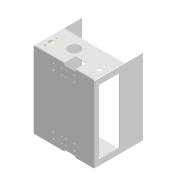
# Autodesk Inventor part: Part75
Saved by Autodesk Inventor 2020.5 (Build 245400000, 400)
## iProperties
Created: 2022-11-22
Part Number: Part75
Material: 一般
Document SubType Name: Sheet Metal
Designer: Administrator
Density: 1 g/cm^3
Appearance: 既定
Sheet Metal Rule: Default_mm
Author: Administrator
Autodesk Inventor part; units mm, degrees
ref_plane "YZ Plane" through (0, 0, 0) normal (1, 0, 0) x (0, 1, 0)
ref_plane "XZ Plane" through (0, 0, 0) normal (0, 1, 0) x (-1, 0, 0)
ref_plane "XY Plane" through (0, 0, 0) normal (0, 0, 1) x (1, 0, 0)
sketch "スケッチ1" plane through (0, 0, 0) normal (0, 0, 1) x (1, 0, 0)
  line L0 (28.4497, -88.6) -> (28.4497, -86) projected
  line L1 (28.4497, -86) -> (31.4997, -86) projected
  line L2 (31.5, -45.4) -> (31.4997, -86) projected
  line L3 (2, -45.3998) -> (31.5, -45.4) projected
  line L4 (2, -45.3998) -> (1.9997, -85.9998) projected
  line L5 (1.9997, -85.9998) -> (5.0497, -85.9998) projected
  line L6 (5.0497, -85.9998) -> (5.0497, -88.5998) projected
  line L7 (28.4497, -88.6) -> (5.0497, -88.5998) projected
  circle A0 centre (27.9998, -75) radius 1.35 projected
  circle A1 centre (5.4999, -58.9999) radius 1.35 projected
  circle A2 centre (5.4998, -74.9999) radius 1.35 projected
  circle A3 centre (27.9999, -59) radius 1.35 projected
  line L8 (38.5497, -88.6) -> (61.9497, -88.6002) projected
  line L9 (61.9497, -86.0002) -> (61.9497, -88.6002) projected
  line L10 (64.9997, -86.0002) -> (61.9497, -86.0002) projected
  line L11 (65, -45.4002) -> (64.9997, -86.0002) projected
  line L12 (65, -45.4002) -> (35.5, -45.4) projected
  line L13 (35.5, -45.4) -> (35.4997, -86) projected
  line L14 (38.5497, -86) -> (35.4997, -86) projected
  line L15 (38.5497, -88.6) -> (38.5497, -86) projected
  circle A4 centre (61.4999, -59.0001) radius 1.35 projected
  circle A5 centre (38.9998, -75) radius 1.35 projected
  circle A6 centre (61.4998, -75.0001) radius 1.35 projected
  circle A7 centre (38.9999, -59) radius 1.35 projected
  line L16 (28.4492, -179.4) -> (28.4492, -182) projected
  line L17 (28.4492, -179.4) -> (5.0492, -179.3998) projected
  line L18 (5.0492, -181.9998) -> (5.0492, -179.3998) projected
  line L19 (1.9992, -181.9998) -> (5.0492, -181.9998) projected
  line L20 (1.999, -222.5998) -> (1.9992, -181.9998) projected
  line L21 (1.999, -222.5998) -> (31.499, -222.6) projected
  line L22 (31.499, -222.6) -> (31.4992, -182) projected
  line L23 (28.4492, -182) -> (31.4992, -182) projected
  circle A8 centre (27.9992, -193) radius 1.35 projected
  circle A9 centre (5.4991, -208.9999) radius 1.35 projected
  circle A10 centre (5.4992, -192.9999) radius 1.35 projected
  circle A11 centre (27.9991, -209) radius 1.35 projected
  line L24 (38.5492, -179.4) -> (61.9492, -179.4002) projected
  line L25 (38.5492, -179.4) -> (38.5492, -182) projected
  line L26 (38.5492, -182) -> (35.4992, -182) projected
  line L27 (35.499, -222.6) -> (35.4992, -182) projected
  line L28 (64.999, -222.6002) -> (35.499, -222.6) projected
  line L29 (64.999, -222.6002) -> (64.9992, -182.0002) projected
  line L30 (64.9992, -182.0002) -> (61.9492, -182.0002) projected
  line L31 (61.9492, -182.0002) -> (61.9492, -179.4002) projected
  circle A12 centre (61.4991, -209.0001) radius 1.35 projected
  circle A13 centre (38.9992, -193) radius 1.35 projected
  circle A14 centre (61.4992, -193.0001) radius 1.35 projected
  circle A15 centre (38.9991, -209) radius 1.35 projected
  line L32 (-44.591, -44.9996) -> (-44.5911, -55.9996) projected
  line L33 (-44.592, -222.9996) -> (-44.5919, -211.9996) projected
  line L34 (111.59, -223.0004) -> (111.5901, -213.0004) projected
  line L35 (111.591, -45.0004) -> (111.5909, -55.0004) projected
  circle A16 centre (61.4992, -193.0001) radius 1.6
  circle A17 centre (61.4991, -209.0001) radius 1.6
  circle A18 centre (38.9992, -193) radius 1.6
  circle A19 centre (38.9991, -209) radius 1.6
  circle A20 centre (27.9992, -193) radius 1.6
  circle A21 centre (27.9991, -209) radius 1.6
  circle A22 centre (5.4991, -208.9999) radius 1.6
  circle A23 centre (5.4992, -192.9999) radius 1.6
  line L36 (-46.4999, -223.01) -> (113.4979, -223.01)
  line L37 (113.4979, -223.01) -> (-46.5009, -223.01)
  line L38 (61.9497, -88.6002) -> (61.9497, -86.0002) projected
  line L39 (61.9497, -88.6002) -> (38.5497, -88.6) projected
  line L40 (38.5497, -86) -> (38.5497, -88.6) projected
  line L41 (35.4997, -86) -> (38.5497, -86) projected
  line L42 (35.5, -45.4) -> (35.4997, -86) projected
  line L43 (35.5, -45.4) -> (65, -45.4002) projected
  line L44 (65, -45.4002) -> (64.9997, -86.0002) projected
  line L45 (61.9497, -86.0002) -> (64.9997, -86.0002) projected
  circle A24 centre (61.4998, -75.0001) radius 1.35 projected
  circle A25 centre (38.9999, -59) radius 1.35 projected
  circle A26 centre (38.9998, -75) radius 1.35 projected
  circle A27 centre (61.4999, -59.0001) radius 1.35 projected
  line L46 (5.0497, -88.5998) -> (28.4497, -88.6) projected
  line L47 (5.0497, -88.5998) -> (5.0497, -85.9998) projected
  line L48 (5.0497, -85.9998) -> (1.9997, -85.9998) projected
  line L49 (2, -45.3998) -> (1.9997, -85.9998) projected
  line L50 (31.5, -45.4) -> (2, -45.3998) projected
  line L51 (31.5, -45.4) -> (31.4997, -86) projected
  line L52 (31.4997, -86) -> (28.4497, -86) projected
  line L53 (28.4497, -86) -> (28.4497, -88.6) projected
  circle A28 centre (27.9999, -59) radius 1.35 projected
  circle A29 centre (5.4998, -74.9999) radius 1.35 projected
  circle A30 centre (27.9998, -75) radius 1.35 projected
  circle A31 centre (5.4999, -58.9999) radius 1.35 projected
  line L54 (35.499, -222.6) -> (113.499, -222.6)
  line L55 (113.499, -222.6) -> (113.499, -45.4)
  line L56 (113.499, -45.4) -> (35.499, -45.4)
  line L57 (35.499, -45.4) -> (35.499, -222.6)
  line L58 (31.499, -222.6) -> (-46.5009, -222.6)
  line L59 (-46.5009, -222.6) -> (-46.5009, -45.4)
  line L60 (-46.5009, -45.4) -> (31.499, -45.4)
  line L61 (31.499, -45.4) -> (31.499, -222.6)
  line L62 (113.499, -45.4) -> (-46.5009, -45.4)
  circle A32 centre (61.4998, -75.0001) radius 1.6
  circle A33 centre (38.9998, -75) radius 1.6
  circle A34 centre (27.9998, -75) radius 1.6
  circle A35 centre (5.4998, -74.9999) radius 1.6
  circle A36 centre (61.4999, -59.0001) radius 1.6
  circle A37 centre (38.9999, -59) radius 1.6
  circle A38 centre (27.9999, -59) radius 1.6
  dimension "d4" = 78
  dimension "d5" = 78
  dimension "d14" = 3.2
  dimension "d15" = 3.2
  dimension "d16" = 3.2
  dimension "d17" = 3.2
  dimension "d18" = 3.2
  dimension "d19" = 3.2
  dimension "d20" = 3.2
  dimension "d21" = 3.2
  dimension "d99" = 78
  dimension "d100" = 3.2
  dimension "d101" = 3.2
  dimension "d102" = 3.2
  dimension "d103" = 3.2
  dimension "d104" = 3.2
  dimension "d105" = 3.2
  dimension "d106" = 3.2
  constraints: 22 end point, 15 centre point, 15 coincident, 4 horizontal, 4 parallel, 2 perpendicular, 1 collinear, 1 point on line
  measures "d4" distance of L27.start L36.end
  measures "d5" distance of L21.end L36.start
  measures "d14" diameter of A16
  measures "d15" diameter of A17
  measures "d16" diameter of A18
  measures "d17" diameter of A19
  measures "d18" diameter of A20
  measures "d19" diameter of A21
  measures "d20" diameter of A22
  measures "d21" diameter of A23
  measures "d99" distance of L56.end L55.end
  measures "d100" diameter of A32
  measures "d101" diameter of A33
  measures "d102" diameter of A34
  measures "d103" diameter of A35
  measures "d104" diameter of A36
  measures "d105" diameter of A37
  measures "d106" diameter of A38
sketch "スケッチ2" plane through (0, 0, 0) normal (0, 1, 0) x (-1, 0, 0)
  point P0 (0, 0)
extrude "押し出し1" add sketch "スケッチ1" along normal blind 1 contours L7 L6 L5 L4 L3 L2 L1 L0 | A0 | A1 | A2 | A3 | L15 L14 L13 L12 L11 L10 L9 L8 | A4 | A5 | A6 | A7 | A32 | A33 | A34 | A35 | A36 | A37 | A38
ref_plane "作業平面1" through (-47.4989, -223.01, -128) normal (-1, -0.0000053, 0) x (0, 0, 1)
sketch "スケッチ8" plane through (-47.4989, -223.01, -128) normal (-1, -0.0000053, 0) x (0, 0, 1)
  line L0 (69.5, 180.01) -> (69.5, 30.01) projected
  line L1 (69.5, 30.01) -> (109.5, 30.01) projected
  line L2 (109.5, 180.01) -> (109.5, 30.01) projected
  line L3 (69.5, 180.01) -> (109.5, 180.01) projected
  line L4 (0, 202.61) -> (127, 202.61) projected
  line L5 (127, 0) -> (0, 0) projected
  ellipse E0 centre (98, 9.01) end of major axis (109, 9.01) minor radius 0.0001 projected
  line L6 (62, 15) -> (117, 15)
  line L7 (117, 15) -> (117, 187.61)
  line L8 (117, 187.61) -> (62, 187.61)
  line L9 (62, 187.61) -> (62, 15)
  line L10 (127, 1) -> (127, 201.61) projected
  point P0 (128, 223.0098)
  dimension "d72" = 55
  dimension "d74" = 202.61
  dimension "d75" = 15
  dimension "d76" = 10
  dimension "d85" = 15
  constraints: 8 end point, 2 parallel, 1 horizontal, 1 perpendicular
  measures "d72" distance of L8.end L7.end
  measures "d74" distance between parallel lines of L4 L5
  measures "d75" distance between parallel lines of L6 L5
  measures "d76" distance between parallel lines of L10 L7
  measures "d85" distance between parallel lines of L4 L8
extrude "押し出し3" cut sketch "スケッチ8" against normal through all both and the other way through all contours L3 L2 L1 L0 | L9 L8 L7 L6
sketch "スケッチ9" plane through (-46.5, -18.4, -1) normal (0, 1, 0) x (1, 0, 0)
  circle A0 centre (13.909, 13.5) radius 2.5 projected
  circle A1 centre (13.909, 44.5) radius 2.5 projected
  circle A2 centre (13.909, 29) radius 11 projected
  line L0 (0.909, 13.8013) -> (0.909, 44.1987) projected
  arc A3 (0.909, 13.8013) -> (26.909, 13.8013) centre (13.909, 29) ccw projected
  line L1 (26.909, 44.1987) -> (26.909, 13.8013) projected
  arc A4 (26.909, 44.1987) -> (0.909, 44.1987) centre (13.909, 29) ccw projected
  circle A5 centre (13.909, 29) radius 4.5 projected
  circle A6 centre (62.25, 43.75) radius 13 projected
  circle A7 centre (95.75, 12.75) radius 12.8 projected
  circle A8 centre (144.091, 13.5) radius 2.5 projected
  circle A9 centre (144.091, 44.5) radius 2.5 projected
  circle A10 centre (144.091, 29) radius 11 projected
  line L2 (157.091, 13.8013) -> (157.091, 44.1987) projected
  arc A11 (157.091, 44.1987) -> (131.091, 44.1987) centre (144.091, 29) ccw projected
  line L3 (131.091, 44.1987) -> (131.091, 13.8013) projected
  arc A12 (131.091, 13.8013) -> (157.091, 13.8013) centre (144.091, 29) ccw projected
  circle A13 centre (62.25, 43.75) radius 15
  circle A14 centre (95.75, 12.75) radius 15
  circle A15 centre (13.909, 29) radius 6
  circle A16 centre (144.091, 29) radius 6
  line L4 (95.75, 12.75) -> (95.75, -2.25)
  line L5 (95.75, 12.75) -> (80.75, 12.75)
  line L6 (159.9989, 0) -> (0.0011, 0) projected
  line L7 (80.75, 0) -> (80.75, 12.75)
  line L8 (95.75, 12.75) -> (110.75, 12.75)
  line L9 (110.75, 0) -> (110.75, 12.75)
  line L10 (80.75, 0) -> (110.75, 0)
  line L11 (80.75, 12.75) -> (110.75, 12.75)
  line L12 (110.75, 12.75) -> (110.75, 27.75)
  line L13 (110.75, 27.75) -> (80.75, 27.75)
  line L14 (80.75, 27.75) -> (80.75, 12.75)
  point P0 (46.5, -1)
  point P1 (95.75, 27.75)
  dimension "d32" = 4
  dimension "d33" = 1
  dimension "d34" = 1
  dimension "d79" = 30
  dimension "d80" = 30
  dimension "d81" = 12
  dimension "d82" = 12
  dimension "d90" = 30
  constraints: 20 end point, 4 centre point, 4 coincident, 3 perpendicular, 3 point on circle, 3 point on line, 2 horizontal, 2 parallel, 2 tangent, 1 collinear, 1 vertical
  measures "d79" diameter of A13
  measures "d80" diameter of A14
  measures "d81" diameter of A15
  measures "d82" diameter of A16
  measures "d90" distance of L13.end L12.end
extrude "押し出し4" [suppressed]
sketch "スケッチ10" plane through (0, 0, 1) normal (0, 0, 1) x (1, 0, 0)
  line L0 (34.25, -18.4) -> (64.25, -18.4) projected
  line L1 (34.25, -18.4) -> (64.25, -18.4)
  line L2 (64.25, -18.4) -> (64.25, -23.4)
  line L3 (64.25, -23.4) -> (34.25, -23.4)
  line L4 (34.25, -23.4) -> (34.25, -18.4)
  line L5 (64.25, -225.01) -> (34.25, -225.01) projected
  line L6 (64.25, -225.01) -> (34.25, -225.01) projected
  line L7 (34.25, -225.01) -> (64.25, -225.01)
  line L8 (64.25, -225.01) -> (64.25, -220.01)
  line L9 (64.25, -220.01) -> (34.25, -220.01)
  line L10 (34.25, -220.01) -> (34.25, -225.01)
  point P0 (0, 0)
  dimension "d94" = 5
  dimension "d95" = 5
  constraints: 16 end point, 4 parallel, 2 horizontal, 2 perpendicular
  measures "d94" distance of L1.end L2.end
  measures "d95" distance of L8.end L7.end
extrude "押し出し5" cut sketch "スケッチ10" against normal blind 10
fillet "フィレット1" [suppressed]
fillet "フィレット2" [suppressed]
fillet "フィレット3" [suppressed]
sketch "スケッチ3" plane through (114.4989, -223.01, -1) normal (1, -0.0000053, 0) x (0.0000053, 1, 0)
  line L0 (202.61, 0) -> (0, 0)
  line L1 (0, 0) -> (0, -128)
  line L2 (0, -128) -> (202.61, -128)
  line L3 (202.61, -128) -> (202.61, 0)
  constraints: 6 end point, 1 horizontal, 1 perpendicular, 1 vertical
sketch "スケッチ6" plane through (113.5, -19.4, -1) normal (0, 1, 0) x (-1, 0, 0)
  line L0 (160, 0) -> (0, 0)
  line L1 (0, 0) -> (0, -78)
  line L2 (0, -78) -> (160, -78)
  line L3 (160, -78) -> (160, 0)
  constraints: 6 end point, 1 horizontal, 1 perpendicular, 1 vertical
equation "\"d32\" = CornerReliefSize"
equation "\"d33\" = GapSize"
equation "\"d34\" = JacobiRadiusSize"
equation "\"BendRadius\" = Thickness"
equation "\"BendReliefWidth\" = Thickness"
equation "\"BendReliefDepth\" = 0.5 * Thickness"
equation "\"CornerReliefSize\" = 4 * Thickness"
equation "\"MinimumRemnant\" = 2 * Thickness"
equation "\"TransitionRadius\" = BendRadius"
equation "\"JacobiRadiusSize\" = BendRadius"
equation "\"GapSize\" = Thickness"
equation "\"Thickness\" = 1"
